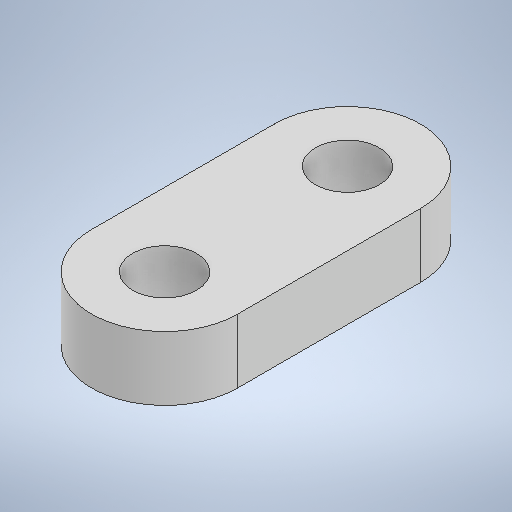
# Autodesk Inventor part: Direccion2,pero3.0
Saved by Autodesk Inventor 2025.2 (Build 292293000, 293)
## iProperties
Created: 2025-03-24
Part Number: Direccion2,pero3.0
Material: Genérico
Document SubType Name: Modeling
Designer: Gabi
Density: 1 g/cm^3
Appearance: Valor por defecto
Author: Gabi
Autodesk Inventor part; units mm, degrees
ref_plane "YZ Plane" through (0, 0, 0) normal (1, 0, 0) x (0, 1, 0)
ref_plane "XZ Plane" through (0, 0, 0) normal (0, 1, 0) x (-1, 0, 0)
ref_plane "XY Plane" through (0, 0, 0) normal (0, 0, 1) x (1, 0, 0)
sketch "Boceto1" plane through (0, 0, 0) normal (0, 1, 0) x (-1, 0, 0)
  circle A0 centre (0, 0) radius 1.75
  arc A1 (4, 0) -> (-4, 0) centre (0, 0) ccw
  line L0 (4, 0) -> (4, -10)
  line L1 (-4, 0) -> (-4, -10)
  line L2 (4, -5) -> (0, -5)
  circle A2 centre (0, -10) radius 1.75
  arc A3 (-4, -10) -> (4, -10) centre (0, -10) ccw
  dimension "d0" = 3.5
  dimension "d1" = 8
  dimension "d2" = 10
  constraints: 6 end point, 4 centre point, 4 point on circle, 3 coincident, 2 symmetric about line, 2 vertical, 1 horizontal, 1 midpoint, 1 tangent, 2 other
  measures "d0" diameter of A0
  measures "d1" diameter of A1
  measures "d2" distance of L0.start L0.end
extrude "Extrusión1" add sketch "Boceto1" along normal blind 3.5
